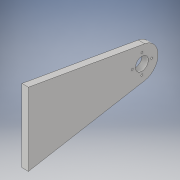
# Autodesk Inventor part: halter_seite
Saved by Autodesk Inventor 2017 (Build 210142000, 142)
## iProperties
Part Number: halter_seite
Material: Generisch
Document SubType Name: Modeling
Designer: Fabio
Density: 1 g/cm^3
Appearance: Vorgabe
Author: Fabio
Autodesk Inventor part; units mm, degrees
ref_plane "YZ Plane" through (0, 0, 0) normal (1, 0, 0) x (0, 1, 0)
ref_plane "XZ Plane" through (0, 0, 0) normal (0, 1, 0) x (-1, 0, 0)
ref_plane "XY Plane" through (0, 0, 0) normal (0, 0, 1) x (1, 0, 0)
sketch "Skizze1" plane through (0, 0, 0) normal (1, 0, 0) x (0, 1, 0)
  arc A0 (200, 0) -> (179.3412, 24.6202) centre (175, 0) ccw
  line L0 (175, 0) -> (179.3412, 24.6202) construction
  line L1 (175, 0) -> (200, 0) construction
  line L2 (179.3412, 24.6202) -> (0, 56.2429)
  line L3 (0, 56.2429) -> (0, 0)
  arc A1 (179.3412, -24.6202) -> (200, 0) centre (175, 0) ccw
  line L4 (179.3412, -24.6202) -> (0, -56.2429)
  line L5 (0, -56.2429) -> (0, 0)
  dimension "d21" = 80
  dimension "d22" = 80
  dimension "d23" = 200
  dimension "d24" = 25
  dimension "d47" = 56.2429
  dimension "d48" = 56.2429
  constraints: 12 end point, 4 point on circle, 2 centre point, 2 symmetric about line, 1 coincident, 1 vertical, 1 other
  measures "d21" angle of L1 L0
  measures "d22" angle of L3 L2
  measures "d23" distance of point (0, 0) L1.end
  measures "d24" radius of A0
  measures "d47" distance of L2.end L3.end
  measures "d48" distance of L4.end L3.end
extrude "Extrusion1" add sketch "Skizze1" along normal blind 10
sketch "Skizze3" plane through (10, 0, 0) normal (1, 0, 0) x (0, 0, -1)
  arc A0 (24.6202, 179.3412) -> (-24.6202, 179.3412) centre (0, 175) ccw projected
  point P0 (0, 0)
  constraints: 1 coincident
hole "Bohrung2" at (10, 175, 0) direction (-1, 0, 0) diameter 20 end through all
sketch "Skizze4" plane through (10, 0, 0) normal (1, 0, 0) x (0, 0, -1)
  arc A0 (24.6202, 179.3412) -> (-24.6202, 179.3412) centre (0, 175) ccw projected
  line L0 (56.2429, 0) -> (24.6202, 179.3412) projected
  line L1 (0, 0) -> (0, 160) construction
  point P0 (15, 175)
  point P1 (0, 190)
  point P2 (-15, 175)
  dimension "d34" = 15
  dimension "d38" = 360
  constraints: 2 end point, 1 vertical, 5 other
  measures "d34" distance of L1.end A0.centre
hole "Bohrung3" at (10, 160, 0) at (10, 175, -15) at (10, 190, 0) at (10, 175, 15) direction (-1, 0, 0) diameter 3 end through all
